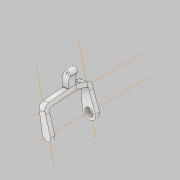
# Autodesk Inventor part: LegRightLarge
Saved by Autodesk Inventor 2019.2 (Build 232265000, 265)
## iProperties
Created: 2019-01-17
Part Number: LegRightLarge
Material: ABS-Kunststoff
Document SubType Name: Modeling
Designer: Lion
Density: 1.06 g/cm^3
Appearance: Weiß
Mass: 2.17468 g
Surface Area: 21.5892 cm^2
Volume: 2.05159 cm^3
Author: Lion
## iProperties of the stored document LegBottom_3D-Druck.ipt
Created: 2019-04-11
Part Number: LegBottom_3D-Druck
Material: Generisch
Document SubType Name: Modeling
Designer: Lion
Density: 1 g/cm^3
Appearance: Vorgabe
Author: Lion
Autodesk Inventor part; units mm, degrees
derived "LegBase.ipt"
sketch "Skizze6" plane through (0, 0, -38.5) normal (0, 0, 1) x (1, 0, 0)
  circle A0 centre (-5.5, 0) radius 1
  arc A1 (-4.2877, 3.2834) -> (-8.555, 1.7078) centre (-5.5, 0) ccw
  line L0 (-5.5, 0) -> (-8.828, 14.6262) construction
  line L1 (-16.355, 12.9135) -> (-1.3009, 16.3388) construction
  circle A2 centre (-16.355, 12.9135) radius 15.4389 construction
  circle A3 centre (-1.3009, 16.3388) radius 15.4389 construction
  line L2 (-8.828, 14.6262) -> (-11.7944, 27.6634) construction
  circle A4 centre (-8.828, 14.6262) radius 2
  line L3 (-6.2928, 15.203) -> (-2.445, -1.7078) construction
  arc A5 (-3.4846, 2.8615) -> (-4.2877, 3.2834) centre (-5.5, 0) ccw
  arc A6 (-8.555, 1.7078) -> (-3.4846, 2.8615) centre (-5.5, 0) ccw
  line L4 (-11.3632, 14.0493) -> (-7.5154, -2.8615) construction
  line L5 (-10.7969, 14.2749) -> (-8.555, 1.7078)
  line L6 (-6.9009, 15.1614) -> (-3.4846, 2.8615)
  line L7 (-10.6339, -1.973) -> (-21, 25) construction
  line L8 (-2, 25) -> (-0.0178, 0.4425) construction
sketch "Skizze2" plane through (0, 0, 0) normal (0, 0, 1) x (1, 0, 0)
  arc A0 (-8.555, 1.7078) -> (-3.4846, 2.8615) centre (-5.5, 0) ccw projected
  circle A1 centre (-5.5, 0) radius 1 projected
  line L0 (-6.9009, 15.1614) -> (-3.4846, 2.8615) projected
  line L1 (-10.7969, 14.2749) -> (-8.555, 1.7078) projected
  circle A2 centre (-8.828, 14.6262) radius 2 projected
  line L2 (-5.5, 0) -> (-8.828, 14.6262) construction
  arc A3 (-12.2407, 13.8496) -> (-11.4713, 16.9202) centre (-8.828, 14.6262) ccw construction
  arc A4 (-11.4713, 16.9202) -> (-12.2407, 13.8496) centre (-8.828, 14.6262) ccw construction
  arc A5 (-0.1371, 1.2203) -> (-4.1723, 5.3373) centre (-5.5, 0) ccw construction
  line L3 (-12.2407, 13.8496) -> (-5.4152, 15.4027)
  line L4 (-12.2407, 13.8496) -> (-5.4152, 15.4027)
  line L5 (-5.8589, 17.3528) -> (-12.6845, 15.7998)
  line L6 (-10.8629, -1.2203) -> (-0.1371, 1.2203) construction
  arc A6 (-0.1371, 1.2203) -> (-10.8629, -1.2203) centre (-5.5, 0) ccw construction
  line L7 (-12.2407, 13.8496) -> (-10.8629, -1.2203)
  line L8 (-0.1371, 1.2203) -> (-5.4152, 15.4027)
  arc A7 (-10.8629, -1.2203) -> (-0.1371, 1.2203) centre (-5.5, 0) ccw
  line L9 (-12.2407, 13.8496) -> (-12.6845, 15.7998)
  line L10 (-5.4152, 15.4027) -> (-5.8589, 17.3528)
  point P0 (0, 0)
  dimension "base_length" = 15
  dimension "r_min" = 7
  dimension "d100" = 2
  dimension "d230" = 11
  constraints: 18 end point, 11 point on circle, 5 centre point, 3 coincident, 3 parallel, 2 perpendicular, 2 point on line, 2 tangent, 1 collinear, 1 midpoint
  measures "base_length" distance of L2.start L2.end
  measures "r_min" diameter of A3
  measures "d100" distance of L5.start L3.end
  measures "d230" diameter of A6
extrude "Extrusion1" add sketch "Skizze2" along normal blind 3.5
extrude "Extrusion22" cut sketch "Skizze2" along normal blind 1.5 contours L1 A2 L0 A0 | L3 A2 | L1 A2 L0 L3 | A1
sketch "Skizze30" plane through (0, 0, 1.5) normal (0, 0, -1) x (-1, 0, 0)
  arc A0 (3.4846, 2.8615) -> (8.555, 1.7078) centre (5.5, 0) ccw projected
  circle A1 centre (5.5, 0) radius 3.5
  point P0 (0, 0)
  constraints: 1 centre point, 1 coincident, 1 concentric
extrude "Extrusion23" cut sketch "Skizze30" against normal up to surface (2 mm away)
ref_plane "Arbeitsebene43" through (0, 0, 35.5) normal (0, 0, 1) x (1, 0, 0)
ref_plane "Arbeitsebene44" through (0, 0, 15) normal (0, 0, 1) x (1, 0, 0)
ref_plane "Arbeitsebene45" through (-8.828, 14.6262, 0) normal (-0.9750777, -0.2218638, 0) x (0, 0, 1)
ref_plane "Arbeitsebene46" through (0, 0, 1.75) normal (0, 0, 1) x (1, 0, 0)
sketch "Skizze58" plane through (0, 0, 35.5) normal (0, 0, 1) x (1, 0, 0)
  circle A0 centre (-5.5, 0) radius 3.5 construction
  line L0 (-15.734, 44.9776) -> (-1.2784, -18.5535) construction
  circle A1 centre (-5.5, 0) radius 3.5
  line L1 (-5.8589, 17.3528) -> (-12.6845, 15.7998) construction
  arc A2 (-8.555, 1.7078) -> (-3.4846, 2.8615) centre (-5.5, 0) ccw projected
  line L2 (-8.9128, -0.7765) -> (-11.2657, 14.0715)
  line L3 (-2.0872, 0.7765) -> (-6.3903, 15.1808)
  line L4 (-11.2657, 14.0715) -> (-11.7094, 16.0217)
  line L5 (-6.3903, 15.1808) -> (-6.834, 17.131)
  line L6 (-11.2657, 14.0715) -> (-6.834, 17.131) construction
  line L7 (-6.3903, 15.1808) -> (-11.7094, 16.0217) construction
  line L8 (-8.9128, -0.7765) -> (-2.0872, 0.7765) construction
  line L9 (-11.7094, 16.0217) -> (-6.834, 17.131)
  point P0 (0, 0)
  point P1 (-9.0498, 15.6012)
  dimension "d261" = 7
  dimension "d262" = 5
  dimension "d263" = 2
  constraints: 16 end point, 3 parallel, 3 point on line, 2 midpoint, 2 point on circle, 1 centre point, 1 coincident, 1 collinear, 1 perpendicular
  measures "d261" diameter of A1
  measures "d262" distance between parallel lines of L5 L4
  measures "d263" distance from line of L2.end L1
extrude "Extrusion50" add sketch "Skizze58" along normal blind 3.5 contours A1 L2 L3 | A1 L2 L4 L9 L5 L3
ref_plane "Arbeitsebene47" through (0, 0, 37.25) normal (0, 0, -1) x (-1, 0, 0)
ref_plane "Arbeitsebene48" through (-8.828, 14.6262, 35.5) normal (-0.9750777, -0.2218638, 0) x (0, 0, 1)
ref_plane "Arbeitsebene57" through (-5.2293, -1.1898, 1.75) normal (-0.9750777, -0.2218638, 0) x (0.2218638, -0.9750777, 0)
sketch "Skizze61" plane through (-12.2407, 13.8496, 0) normal (-0.9750777, -0.2218638, 0) x (0, 0, 1)
  arc A0 (3.3685, 6.3554) -> (0, 2) centre (4.5, 2) ccw
  arc A1 (4.2486, 2.9679) -> (3.5, 2) centre (4.5, 2) ccw
  line L0 (0, 2) -> (3.5, 2)
  line L1 (4.2486, 2.9679) -> (9.2486, 4.2668)
  line L2 (9.2486, 4.2668) -> (8.3685, 7.6544)
  line L3 (8.3685, 7.6544) -> (3.3685, 6.3554)
  line L4 (0, 2) -> (3.5, 2) construction
  line L5 (35.5, 2) -> (39, 2) construction
  line L6 (3.5, 2) -> (4.5, 2) construction
  arc A2 (12, 8) -> (8.3685, 7.6544) centre (11.2601, -3.4762) ccw
  arc A3 (12, 4.4895) -> (9.2486, 4.2668) centre (11.2601, -3.4762) ccw
  line L7 (11.2601, -3.4762) -> (9.2486, 4.2668) construction
  line L8 (12, 4.4895) -> (12, 8)
  line L9 (15, 31.1272) -> (15, -34.0277) construction
  arc A4 (39, 2) -> (34.9063, 6.4816) centre (34.5, 2) ccw
  arc A5 (35.5, 2) -> (34.5903, 2.9959) centre (34.5, 2) ccw
  line L10 (35.5, 2) -> (34.5, 2) construction
  line L11 (34.5903, 2.9959) -> (18, 4.5)
  line L12 (18.316, 7.9857) -> (34.9063, 6.4816)
  arc A6 (18.316, 7.9857) -> (18, 8) centre (18, 4.5) ccw
  line L13 (18, 4.5) -> (18, 8)
  line L14 (35.5, 2) -> (39, 2)
  line L15 (18, 8) -> (12, 8) construction
  point P0 (0, -16.2203)
  dimension "d280" = 3
  dimension "d281" = 6
  dimension "d282" = 1
  dimension "d283" = 8
  dimension "d284" = 5
  dimension "d285" = 3
  dimension "d286" = 1
  constraints: 26 end point, 15 point on circle, 7 centre point, 5 coincident, 5 tangent, 3 collinear, 3 perpendicular, 2 horizontal, 2 vertical, 1 parallel
  measures "d280" distance between parallel lines of L9 L8
  measures "d281" distance from line of L8.end L0
  measures "d282" distance of L0.end L6.end
  measures "d283" distance from line of A2.centre L1
  measures "d284" horizontal distance of L2.end L3.end
  measures "d285" distance between parallel lines of L9 L13
  measures "d286" distance of L5.start L10.end
extrude "Extrusion51" add sketch "Skizze61" against normal up to surface (7 mm away) contours L3 L2 L1 A1 L0 A0 | A2 L8 A3 L2
extrude "Extrusion52" add sketch "Skizze61" against normal up to surface (5 mm away) from surface at -1 contours L14 A5 L11 L13 A6 L12 A4
sketch "Skizze62" plane through (-7.3887, 19.5687, 18) normal (0, 0, -1) x (-0.9750777, -0.2218638, 0)
  line L0 (0, 3.5) -> (0, 0) projected
  line L1 (5, 0) -> (0, 0) projected
  line L2 (5, 0) -> (5, 3.5) projected
  line L3 (5, 3.5) -> (0, 3.5) projected
  point P0 (-2.8629, -20.7203)
extrude "Extrusion53" add sketch "Skizze62" along normal up to next
chamfer "Fase13" distance 1 distance2 8 1 edges at (-6.8007, 21.4918, 12) measured on face at (-7.2882, 21.3809, 12)
chamfer "Fase14" distance 1 distance2 8 1 edges at (-13.6262, 19.9388, 12) measured on face at (-13.1387, 20.0497, 12)
ref_plane "Arbeitsebene59" through (-5.5, 0, 0) normal (0.54198, -0.8403914, 0) x (0, 0, 1)
ref_plane "Arbeitsebene58" through (-5.5, 0, 0) normal (-0.8403914, -0.54198, 0) x (0, 0, 1)
sketch "Skizze63" plane through (0, 0, 15) normal (0, 0, 1) x (1, 0, 0)
  line L0 (-13.0406, 21.8721) -> (-8.1652, 22.9814) construction
  line L1 (-13.0406, 21.8721) -> (-8.1652, 22.9814) construction
  line L2 (-1.2784, -18.5535) -> (-15.734, 44.9776) construction
  arc A0 (-11.5927, 34.0499) -> (-13.0406, 21.8721) centre (4.7842, 25.9279) ccw
  arc A1 (-7.1134, 31.8284) -> (-8.1652, 22.9814) centre (4.7842, 25.9279) ccw
  line L3 (-13.0406, 21.8721) -> (-8.1652, 22.9814)
  line L4 (-7.1134, 31.8284) -> (-6.9138, 32.2307)
  line L5 (-6.9138, 32.2307) -> (-11.3932, 34.4522)
  line L6 (-11.3932, 34.4522) -> (-11.5927, 34.0499)
  line L7 (-8.1652, 22.9814) -> (4.7842, 25.9279) construction
  arc A2 (-6.9138, 32.2307) -> (-11.3932, 34.4522) centre (-9.1535, 33.3414) ccw
  circle A3 centre (-9.1535, 33.3414) radius 1.05
  line L8 (38.6014, 28.4416) -> (-37.4382, -20.5974) construction
  line L9 (9.8469, -23.7968) -> (-39.666, 52.9777) construction
  point P0 (0, 0)
  dimension "d301" = 2.1
  dimension "d304" = 30
  dimension "d305" = 15
  dimension "d312" = 12.9494
  constraints: 10 end point, 6 point on circle, 4 centre point, 3 coincident, 2 tangent, 1 collinear, 1 midpoint, 1 parallel, 1 perpendicular
  measures "d301" diameter of A3
  measures "d304" distance from line of L8 A2.centre
  measures "d305" distance from line of point (-9.154, 33.341) L9
  measures "d312" horizontal distance of L0.end L7.end
extrude "Extrusion54" add sketch "Skizze63" along normal mid plane 6
sketch "Skizze64" plane through (0, 0, 18) normal (0, 0, 1) x (1, 0, 0)
  circle A0 centre (-9.1535, 33.3414) radius 1.05 projected
  point P0 (0, 0)
extrude "Extrusion55" cut sketch "Skizze64" against normal up to next
fillet "Rundung37" [suppressed]
fillet "Rundung38" [suppressed]
fillet "Rundung39" [suppressed]
